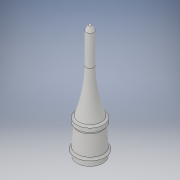
# Autodesk Inventor part: B
Saved by Autodesk Inventor 2017 (Build 210142000, 142)
## iProperties
Part Number: B
Material: 一般
Document SubType Name: Modeling
Designer: user
Density: 1 g/cm^3
Appearance: 預設
Author: user
Autodesk Inventor part; units mm, degrees
ref_plane "YZ Plane" through (0, 0, 0) normal (1, 0, 0) x (0, 1, 0)
ref_plane "XZ Plane" through (0, 0, 0) normal (0, 1, 0) x (-1, 0, 0)
ref_plane "XY Plane" through (0, 0, 0) normal (0, 0, 1) x (1, 0, 0)
sketch "草圖2" plane through (0, 0, 0) normal (0, 0, 1) x (1, 0, 0)
  line L0 (0, 0) -> (17, 0)
  line L1 (17, 0) -> (19.5, 8)
  line L2 (19.5, 8) -> (17.5, 8)
  line L3 (17.5, 8) -> (15.5, 39)
  line L4 (15.5, 39) -> (17.5, 39)
  line L5 (17.5, 39) -> (17.5, 44)
  line L6 (17.5, 44) -> (15.5, 44)
  line L7 (0, 0) -> (0, 150)
  line L8 (1.7565, 148.9565) -> (5, 143)
  line L9 (5, 143) -> (5, 103)
  arc A0 (5, 103) -> (15.5, 44) centre (194.97, 106.3739) ccw
  line L10 (0, 0) -> (-19.5, 0) construction
  arc A1 (17, 0) -> (0, 5.2901) centre (-1.25, -28.6869) ccw
  line L11 (0, 150) -> (0, 148)
  arc A2 (1.7565, 148.9565) -> (0, 150) centre (0, 148) ccw
  dimension "d2" = 7
  dimension "d3" = 10
  dimension "d4" = 17
  dimension "d5" = 39
  dimension "d6" = 5
  dimension "d7" = 40
  dimension "d8" = 35
  dimension "d9" = 8
  dimension "d10" = 44
  dimension "d11" = 150
  dimension "d12" = 2
  dimension "d13" = 2
  dimension "d15" = 2
  dimension "d16" = 190
  dimension "d20" = 19.5
  dimension "d21" = 34
  dimension "d22" = 142
  dimension "d23" = 2.7099
  dimension "d28" = 4
  dimension "d29" = 61.43
  dimension "d30" = 140
  constraints: 24 end point, 6 point on circle, 3 centre point, 3 point on line, 2 horizontal, 2 parallel, 2 perpendicular, 2 vertical, 1 line through centre, 1 tangent
  measures "d2" vertical distance of L8.end L11.start
  measures "d3" diameter of L8.end L7
  measures "d4" distance of L0.start L0.end
  measures "d5" diameter of L1.end L7
  measures "d6" distance of L4.end L5.end
  measures "d7" distance of L8.end L9.end
  measures "d8" diameter of L5.end L7
  measures "d9" distance from line of L1.end L0
  measures "d10" distance between parallel lines of L6 L0
  measures "d11" distance from line of L11.start L0
  measures "d12" distance of L1.end L2.end
  measures "d13" distance of L4.end L3.end
  measures "d15" distance of L5.end L6.end
  measures "d16" radius of A0
  measures "d20" distance of L0.start L10.end
  measures "d21" radius of A1
  measures "d22" distance from line of L7.end L2
  measures "d23" distance from line of A1.end L2
  measures "d28" diameter of A2
  measures "d29" angle of L8 L2
  measures "d30" distance from line of L11.end L2
revolve "迴轉2" add sketch "草圖2" angle 360 about axis through (0, 0, 0) along (0, 1, 0) contours A1 L7 A2 L8 L9 A0 L6 L5 L4 L3 L2 L1
fillet "圓角3" radius 3 3 edges at (-17.5, 8, 0) (-15.5, 44, 0) (-15.5, 39, 0)
